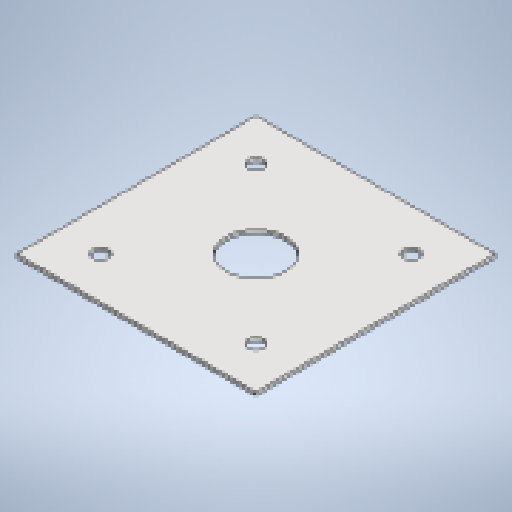
# Autodesk Inventor part: NDM-VOS 111 sredder wall _CPY
Saved by Autodesk Inventor 2025.1 (Build 291241020, 241B)
## iProperties
Created: 2024-11-03
Part Number: NDM-VOS 111 sredder wall _CPY
Material: Stainless Steel
Document SubType Name: Sheet Metal
Designer: user
Mass: 280.619 g
Surface Area: 364.406 cm^2
Volume: 35.0774 cm^3
Density: 8 g/cm^3
Sheet Metal Rule: AISI304 3mm Die 32
Sheet Metal Width: 0,000 mm
Sheet Metal Length: 0,000 mm
Sheet Metal Area: 0,000 mm^2
Appearance: Default
Author: admin
Autodesk Inventor part; units mm, degrees
ref_plane "YZ Plane" through (0, 0, 0) normal (1, 0, 0) x (0, 1, 0)
ref_plane "XZ Plane" through (0, 0, 0) normal (0, 1, 0) x (-1, 0, 0)
ref_plane "XY Plane" through (0, 0, 0) normal (0, 0, 1) x (1, 0, 0)
sketch "Sketch1" plane through (0, 0, 0) normal (0, 0, 1) x (1, 0, 0)
  line L0 (-100, 100) -> (100, 100)
  line L1 (100, 100) -> (100, -100)
  line L2 (100, -100) -> (-100, -100)
  line L3 (-100, -100) -> (-100, 100)
  line L4 (-100, 100) -> (100, -100) construction
  line L5 (100, 100) -> (-100, -100) construction
  point P0 (0, 0)
  point P1 (0, 0)
  point P2 (0, 0)
  dimension "d25" = 200
  dimension "d26" = 200
  measures "d25" distance of L1.end L2.end
  measures "d26" distance of L0.end L1.end
extrude "Plate1" add sketch "Sketch1" along normal blind 3
sketch "Sketch6" plane through (0, 0, 3) normal (0, 0, 1) x (1, 0, 0)
  circle A0 centre (-75, 0) radius 15
  circle A1 centre (75, 0) radius 15
  line L0 (0, 0) -> (0, 55.0725) construction
  dimension "d37" = 30
  dimension "d38" = 150
  constraints: 2 centre point, 2 end point, 1 horizontal alignment, 1 vertical, 1 other
  measures "d37" diameter of A0
  measures "d38" distance of A1.centre A0.centre
cut "Cut1" [suppressed]
sketch "Sketch8" plane through (0, 0, 0) normal (1, 0, 0) x (0, 1, 0)
  line L0 (-94.2929, 40) -> (94.2929, 40) projected
  circle A0 centre (0, 30) radius 6.5
  line L1 (89.2929, 5) -> (-89.2929, 5) projected
  point P0 (0, 0)
  dimension "d48" = 13
  dimension "d49" = 25
  constraints: 1 centre point, 1 vertical alignment
  measures "d48" diameter of A0
  measures "d49" distance from line of L1 A0.centre
extrude "Extrusion3" [suppressed]
pattern_linear "Rectangular Pattern2" [suppressed]
sketch "Sketch9" plane through (0, 0, 3) normal (0, 0, 1) x (1, 0, 0)
  circle A0 centre (-65, 65) radius 6.5
  point P0 (0, 0)
  point P1 (-225, 65)
  dimension "d55" = 13
  dimension "d73" = 65
  dimension "d74" = 65
  constraints: 1 centre point, 1 horizontal alignment
  measures "d55" diameter of A0
  measures "d73" horizontal distance of point (0, 0) A0.centre
  measures "d74" horizontal distance of A0.centre point (0, 0)
extrude "Cut2" cut sketch "Sketch9" against normal blind 3
mirror "Mirror1" about plane through (0, 0, 0) normal (1, 0, 0) of "Cut2"
mirror "Mirror2" about plane through (0, 0, 0) normal (0, 1, 0) of "Cut2", "Mirror1"
sketch "Sketch10" plane through (0, 0, 0) normal (0, 0, -1) x (-1, 0, 0)
  circle A0 centre (0, 0) radius 25
  dimension "d75" = 50
  constraints: 1 centre point, 1 coincident
  measures "d75" diameter of A0
extrude "Cut3" cut sketch "Sketch10" against normal blind 3
equation "\"d74\" = d73"
equation "\"d26\" = Гриндер_высота"
equation "\"d38\" = Гриндер_Валы_между_центрами"
equation "\"d39\" = Thickness"
equation "\"d48\" = Гриндер_диам_отврс_корпуса"
equation "\"d49\" = Гриндер_отступ_отврс_корпуса"
equation "\"d55\" = Гриндер_диам_отврс_корпуса"
equation "\"d57\" = Thickness"
equation "\"d76\" = Thickness"
equation "\"d2\" = Thickness"
equation "\"BendReliefWidth\" = Thickness"
equation "\"BendReliefDepth\" = 0.5 * Thickness"
equation "\"CornerReliefSize\" = 4 * Thickness"
equation "\"MinimumRemnant\" = 2 * Thickness"
equation "\"TransitionRadius\" = BendRadius"
equation "\"JacobiRadiusSize\" = BendRadius"
equation "\"GapSize\" = Thickness"
equation "\"Гриндер_отступ_отврс_корпуса\" = 25"
equation "\"Гриндер_диам_отврс_корпуса\" = 13"
equation "\"Гриндер_высота\" = 200"
equation "\"Гриндер_Валы_между_центрами\" = 150"
equation "\"Thickness\" = 3"
equation "\"BendRadius\" = 5"
body "Solid1"
